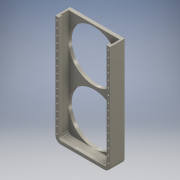
# Autodesk Inventor part: Cup_Dispenser_Hull
Saved by Autodesk Inventor 2016 (Build 200138000, 138)
## iProperties
Created: 2015-07-09
Part Number: Cup_Dispenser_Hull
Material: Generic
Document SubType Name: Modeling
Designer: marku
Density: 1 g/cm^3
Appearance: Titanium
Author: marku
Autodesk Inventor part; units mm, degrees
ref_plane "YZ Plane" through (0, 0, 0) normal (1, 0, 0) x (0, 1, 0)
ref_plane "XZ Plane" through (0, 0, 0) normal (0, 1, 0) x (-1, 0, 0)
ref_plane "XY Plane" through (0, 0, 0) normal (0, 0, 1) x (1, 0, 0)
sketch "Sketch1" plane through (0, 0, 0) normal (0, 1, 0) x (-1, 0, 0)
  line L0 (-50, 100) -> (50, 100)
  line L1 (50, 100) -> (50, -90)
  line L2 (40, -100) -> (-40, -100)
  line L3 (-50, -90) -> (-50, 100)
  line L4 (-50, 100) -> (50, -100) construction
  line L5 (50, 100) -> (-50, -100) construction
  line L6 (-50, 100) -> (50, 100)
  line L7 (50, 100) -> (50, 0)
  line L8 (50, 0) -> (-50, 0)
  line L9 (-50, 0) -> (-50, 100)
  line L10 (50, 0) -> (-50, 100) construction
  line L11 (-50, 0) -> (50, 100) construction
  circle A0 centre (0, 50) radius 47
  line L12 (47, 50) -> (50, 50) construction
  arc A1 (40, -100) -> (50, -90) centre (40, -90) ccw
  arc A2 (-50, -90) -> (-40, -100) centre (-40, -90) ccw
  point P0 (0, 0)
  dimension "d0" = 100
  dimension "d1" = 200
  dimension "d2" = 100
  dimension "d3" = 3
  dimension "d4" = 10
  constraints: 26 end point, 5 point on line, 4 midpoint, 4 parallel, 4 point on circle, 4 tangent, 3 horizontal, 2 centre point, 2 perpendicular, 1 equal radius, 1 horizontal alignment, 2 other
  measures "d0" distance of L4.end L5.end
  measures "d1" distance of L0.end L4.end
  measures "d2" distance between parallel lines of L8 L0
  measures "d3" distance of L12.start L12.end
  measures "d4" radius of A1
extrude "Extrusion1" add sketch "Sketch1" along normal blind 6
sketch "Sketch2" plane through (0, 0, 0) normal (0, -1, 0) x (1, 0, 0)
  circle A0 centre (0, 50) radius 47 construction
  line L0 (50, 100) -> (50, -90) projected
  line L1 (-50, 100) -> (50, 100) projected
  line L2 (-50, -90) -> (-50, 100) projected
  arc A1 (-50, -90) -> (-40, -100) centre (-40, -90) ccw projected
  line L3 (40, -100) -> (-40, -100) projected
  arc A2 (40, -100) -> (50, -90) centre (40, -90) ccw projected
  line L4 (47, -90) -> (47, 97)
  line L5 (47, 97) -> (-47, 97)
  line L6 (-47, 97) -> (-47, -90)
  arc A3 (-47, -90) -> (-40, -97) centre (-40, -90) ccw
  line L7 (-40, -97) -> (40, -97)
  arc A4 (40, -97) -> (47, -90) centre (40, -90) ccw
  line L8 (47, 97) -> (47, 100)
  line L9 (-47, 97) -> (-47, 100)
  point P0 (0, 0)
  dimension "d7" = 3
  constraints: 12 end point, 4 point on circle, 2 centre point, 2 point on line, 1 perpendicular, 1 vertical, 5 other
  measures "d7" distance between parallel lines of L0 L4
extrude "Extrusion2" add sketch "Sketch2" along normal blind 15 contours L0 A2 L3 A1 L2 L1 L9 L6 A3 L7 A4 L4 L8
sketch "Sketch3" plane through (0, -15, 0) normal (0, -1, 0) x (1, 0, 0)
  line L0 (50, -90) -> (50, 100) projected
  line L1 (50, 100) -> (47, 100) projected
  line L2 (47, 100) -> (47, -90) projected
  arc A0 (40, -97) -> (47, -90) centre (40, -90) ccw projected
  line L3 (40, -97) -> (-40, -97) projected
  arc A1 (-47, -90) -> (-40, -97) centre (-40, -90) ccw projected
  line L4 (-47, -90) -> (-47, 100) projected
  line L5 (-47, 100) -> (-50, 100) projected
  line L6 (-50, 100) -> (-50, -90) projected
  arc A2 (-50, -90) -> (-40, -100) centre (-40, -90) ccw projected
  line L7 (-40, -100) -> (40, -100) projected
  arc A3 (40, -100) -> (50, -90) centre (40, -90) ccw projected
  line L8 (47, 100) -> (44, 100)
  line L9 (-50, 100) -> (50, 100) construction
  line L10 (44, 100) -> (44, -90)
  line L11 (40, -94) -> (15, -94)
  arc A4 (40, -94) -> (44, -90) centre (40, -90) ccw
  line L12 (0, 0) -> (0, -136) construction
  line L13 (-47, 100) -> (-44, 100)
  line L14 (-44, 100) -> (-44, -90)
  line L15 (-40, -94) -> (15, -94)
  arc A5 (-44, -90) -> (-40, -94) centre (-40, -90) ccw
  dimension "d10" = 3
  constraints: 14 end point, 4 point on circle, 4 symmetric about line, 2 centre point, 2 parallel, 2 tangent, 1 coincident, 1 point on line, 1 vertical, 1 other
  measures "d10" distance between parallel lines of L2 L10
extrude "Extrusion3" add sketch "Sketch3" along normal blind 6
sketch "Sketch5" plane through (0, 6, 0) normal (0, 1, 0) x (1, 0, 0)
  circle A0 centre (0, -50) radius 47 projected
  line L0 (50, -100) -> (50, 90) projected
  arc A1 (50, 90) -> (40, 100) centre (40, 90) ccw projected
  line L1 (40, 100) -> (-40, 100) projected
  arc A2 (-40, 100) -> (-50, 90) centre (-40, 90) ccw projected
  line L2 (-50, 90) -> (-50, -100) projected
  line L3 (-50, -100) -> (50, -100) projected
  line L4 (-67.6504, 0) -> (67.3496, 0) construction
  circle A3 centre (0, 50) radius 47
  point P0 (0, 0)
  constraints: 2 end point, 1 centre point, 1 horizontal, 1 point on line, 1 symmetric about line, 1 other
extrude "Extrusion4" cut sketch "Sketch5" against normal up to next contours A3
sketch "Sketch6" plane through (0, 6, 0) normal (0, 1, 0) x (1, 0, 0)
  circle A0 centre (0, -50) radius 47 projected
  circle A1 centre (0, 50) radius 47 projected
  circle A2 centre (0, 50) radius 47 projected
  circle A3 centre (0, -50) radius 47 projected
  line L0 (50, -100) -> (50, 90) projected
  arc A4 (50, 90) -> (40, 100) centre (40, 90) ccw projected
  line L1 (40, 100) -> (-40, 100) projected
  arc A5 (-40, 100) -> (-50, 90) centre (-40, 90) ccw projected
  line L2 (-50, 90) -> (-50, -100) projected
  line L3 (-50, -100) -> (50, -100) projected
  line L4 (-50.0326, 0) -> (43.9674, 0) construction
  line L5 (0, -50) -> (-70, -50) construction
  line L6 (0, -50) -> (0, -118) construction
  point P0 (0, 0)
  point P1 (-41, -9)
  point P2 (-41, -91)
  point P3 (41, -9)
  point P4 (41, -91)
  point P5 (-41, 9)
  point P6 (-41, 91)
  point P7 (41, 91)
  point P8 (41, 9)
  dimension "d15" = 18
  dimension "d16" = 9
  constraints: 7 symmetric about line, 6 end point, 2 horizontal, 1 point on line, 1 vertical
  measures "d15" diameter of point (-41, -9) L4
  measures "d16" distance from line of L2 point (-41, -9)
hole "Hole1" at (-41, 6, 9) at (-41, 6, 91) at (41, 6, 91) at (41, 6, 9) at (-41, 6, -91) at (-41, 6, -9) at (41, 6, -91) at (41, 6, -9) direction (0, -1, 0) diameter 3 depth 4 tip angle 118
sketch "Sketch7" plane through (0, -21, 0) normal (0, -1, 0) x (1, 0, 0)
  line L0 (47, 100) -> (47, -90) construction
  line L1 (47, 50) -> (47, 100) projected
  line L2 (47, -50) -> (47, 50) projected
  line L3 (47, -90) -> (47, -50) projected
  line L4 (-47, -90) -> (-47, 100) construction
  line L5 (-47, -50) -> (-47, -90) projected
  line L6 (-47, 50) -> (-47, -50) projected
  line L7 (-47, 100) -> (-47, 50) projected
  line L8 (47, 100) -> (47, -90) projected
  line L9 (0, 119) -> (0, 0) construction
  point P0 (47, 94)
  point P1 (-47, 94)
  point P2 (-47, 82)
  point P3 (47, 82)
  point P4 (-47, 70)
  point P5 (47, 70)
  point P6 (-47, 58)
  point P7 (47, 58)
  point P8 (-47, 46)
  point P9 (47, 46)
  point P10 (-47, 34)
  point P11 (47, 34)
  point P12 (-47, 22)
  point P13 (47, 22)
  point P14 (-47, 10)
  point P15 (47, 10)
  point P16 (-47, -2)
  point P17 (47, -2)
  point P18 (-47, -14)
  point P19 (47, -14)
  point P20 (-47, -26)
  point P21 (47, -26)
  point P22 (-47, -38)
  point P23 (47, -38)
  point P24 (-47, -50)
  point P25 (47, -50)
  point P26 (-47, -62)
  point P27 (47, -62)
  point P28 (-47, -74)
  point P29 (47, -74)
  point P30 (-47, -86)
  point P31 (47, -86)
  dimension "d24" = 6
  dimension "d27" = 12
  constraints: 2 end point, 2 vertical, 1 point on line, 1 symmetric about line, 30 other
  measures "d24" distance of L0.start point (47, 94)
  measures "d27" distance of point (-47, 94) point (-47, 82)
hole "Hole2" at (47, -21, 94) at (-47, -21, 94) at (-47, -21, 82) at (47, -21, 82) at (-47, -21, 70) at (47, -21, 70) at (-47, -21, 58) at (47, -21, 58) at (-47, -21, 46) at (47, -21, 46) at (-47, -21, 34) at (47, -21, 34) at (-47, -21, 22) at (47, -21, 22) at (-47, -21, 10) at (47, -21, 10) at (-47, -21, -2) at (47, -21, -2) at (-47, -21, -14) at (47, -21, -14) at (-47, -21, -26) at (47, -21, -26) at (-47, -21, -38) at (47, -21, -38) at (-47, -21, -50) at (47, -21, -50) at (-47, -21, -62) at (47, -21, -62) at (-47, -21, -74) at (47, -21, -74) at (-47, -21, -86) at (47, -21, -86) direction (0, 1, 0) diameter 3 depth 4 tip angle 118
equation "\"d0\" = hull_width"
equation "\"d1\" = hull_length"
equation "\"d2\" = hull_width"
equation "\"d4\" = roundness"
equation "\"d5\" = 2 * thickness"
equation "\"d7\" = thickness"
equation "\"d8\" = 5 * thickness"
equation "\"d10\" = thickness"
equation "\"d11\" = 2 * thickness"
equation "\"d13\" = 2 * thickness"
equation "\"d15\" = 6 * thickness"
equation "\"d16\" = 3 * thickness"
equation "\"d22\" = 1.33333 * thickness"
equation "\"d24\" = 2 * thickness"
equation "\"d27\" = 4 * thickness"
equation "\"d37\" = 1.33333 * thickness"
equation "\"thickness\" = 3"
equation "\"roundness\" = 10"
equation "\"hull_width\" = 100"
equation "\"hull_length\" = 2 * hull_width"
body "Solid1"
